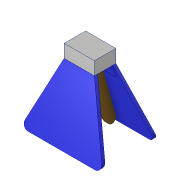
# Autodesk Inventor part: ANTENNA
Saved by Autodesk Inventor 2018 (Build 220112000, 112)
## iProperties
Created: 2020-03-03
Part Number: ANTENNA
Material: Generic
Document SubType Name: Modeling
Designer: nnico
Density: 1 g/cm^3
Appearance: Blue - Wall Paint - Glossy
Author: nnico
Autodesk Inventor part; units mm, degrees
ref_plane "YZ Plane" through (0, 0, 0) normal (1, 0, 0) x (0, 1, 0)
ref_plane "XZ Plane" through (0, 0, 0) normal (0, 1, 0) x (-1, 0, 0)
ref_plane "XY Plane" through (0, 0, 0) normal (0, 0, 1) x (1, 0, 0)
sketch "Sketch1" plane through (0, 0, 0) normal (0, 1, 0) x (-1, 0, 0)
  line L0 (126, -87.5) -> (-126, -87.5)
  line L1 (-126, -87.5) -> (-126, 87.5)
  line L2 (-126, 87.5) -> (126, 87.5)
  line L3 (126, 87.5) -> (126, -87.5)
  line L4 (0, -87.5) -> (0, 87.5) construction
  line L5 (126, 0) -> (-126, 0) construction
  point P0 (0, 0)
  point P1 (0, 0)
  dimension "d0" = 252
  dimension "d1" = 175
  constraints: 12 end point, 5 midpoint, 2 parallel, 1 coincident, 1 horizontal, 1 perpendicular
  measures "d0" distance of L1.end L2.end
  measures "d1" distance of L0.end L1.end
extrude "Extrusion1" add sketch "Sketch1" along normal blind 235
sketch "Sketch3" plane through (0, 235, 0) normal (0, 1, 0) x (1, 0, 0)
  line L0 (126, 87.5) -> (-126, 87.5) projected
  line L1 (-126, 87.5) -> (-126, -87.5) projected
  line L2 (-126, -87.5) -> (126, -87.5) projected
  line L3 (126, -87.5) -> (126, 87.5) projected
  line L4 (-46.5, 33) -> (46.5, 33)
  line L5 (46.5, 33) -> (46.5, -33)
  line L6 (46.5, -33) -> (-46.5, -33)
  line L7 (-46.5, -33) -> (-46.5, 33)
  line L8 (0, 33) -> (0, -33) construction
  line L9 (-46.5, 0) -> (46.5, 0) construction
  point P0 (0, 0)
  point P1 (0, 0)
  dimension "d6" = 93
  dimension "d7" = 66
  constraints: 12 end point, 5 midpoint, 2 parallel, 1 coincident, 1 horizontal, 1 perpendicular
  measures "d6" distance of L5.end L6.end
  measures "d7" distance of L4.end L5.end
extrude "Extrusion2" cut sketch "Sketch3" against normal blind 40
sketch "Sketch4" plane through (-126, 0, 87.5) normal (0, 0, 1) x (1, 0, 0)
  line L0 (79.5, 235) -> (79.5, 195) construction
  line L1 (172.5, 235) -> (172.5, 195) construction
  line L2 (252, 0) -> (0, 0) projected
  line L3 (79.5, 195) -> (0, 0)
  line L4 (172.5, 195) -> (252, 0)
  line L5 (0, 0) -> (0, 195) projected
  line L6 (252, 195) -> (0, 195) projected
  line L7 (252, 0) -> (252, 195) projected
  point P0 (126, 0)
  constraints: 4 end point
extrude "Extrusion3" cut sketch "Sketch4" against normal up to next contours L4 L6 L7 | L5 L6 L3
sketch "Sketch5" plane through (-46.5, 235, -33) normal (-1, 0, 0) x (0, 0, 1)
  line L0 (66, 0) -> (66, -40) projected
  line L1 (120.5, -235) -> (120.5, -40) projected
  line L2 (66, -40) -> (120.5, -235)
  line L3 (120.5, -235) -> (120.5, -40)
  line L4 (120.5, -40) -> (66, -40) projected
  line L5 (120.5, -40) -> (66, -40)
  line L6 (0, -40) -> (-54.5, -40) projected
  line L7 (0, -40) -> (-54.5, -235)
  line L8 (-54.5, -235) -> (-54.5, -40)
  point P0 (33, -235)
  constraints: 10 end point, 2 collinear, 1 vertical
extrude "Extrusion4" cut sketch "Sketch5" along normal up to next
sketch "Sketch6" plane through (-46.5, 235, -33) normal (-1, 0, 0) x (0, 0, 1)
  line L0 (-54.5, -40) -> (0, -40) projected
  line L1 (-54.5, -235) -> (-54.5, -40) projected
  line L2 (-54.5, -235) -> (0, -40) projected
  line L3 (66, -40) -> (120.5, -235) projected
  line L4 (120.5, -40) -> (120.5, -235) projected
  line L5 (66, -40) -> (120.5, -40) projected
  point P0 (33, -235)
extrude "Extrusion5" cut sketch "Sketch6" against normal up to next
sketch "Sketch7" plane through (-46.5, 235, -33) normal (-1, 0, 0) x (0, 0, 1)
  line L0 (66, -40) -> (0, -40) projected
  line L1 (0, -40) -> (10, -40)
  line L2 (0, -40) -> (-54.5, -235) projected
  line L3 (120.5, -235) -> (-54.5, -235) projected
  line L4 (-54.5, -235) -> (-44.5, -235)
  line L5 (-44.5, -235) -> (10, -40)
  line L6 (66, -40) -> (56, -40)
  line L7 (120.5, -235) -> (110.5, -235)
  line L8 (110.5, -235) -> (56, -40)
  line L9 (120.5, -235) -> (66, -40) projected
  point P0 (33, -235)
  dimension "d16" = 10
  dimension "d17" = 10
  dimension "d18" = 10
  dimension "d19" = 10
  constraints: 12 end point, 4 point on line
  measures "d16" distance of L0.end L1.end
  measures "d17" distance of L2.end L4.end
  measures "d18" distance of L0.start L6.end
  measures "d19" distance of L3.start L7.end
extrude "Extrusion6" cut sketch "Sketch7" along normal up to next contours L8 L3 L5 L0
sketch "Sketch8" plane through (-46.5, 235, -33) normal (-1, 0, 0) x (0, 0, 1)
  line L0 (110.5, -235) -> (56, -40) projected
  line L1 (10, -40) -> (-44.5, -235) projected
  line L2 (56, -40) -> (10, -40)
  line L3 (110.5, -235) -> (-44.5, -235) projected
  point P0 (33, -235)
  constraints: 2 end point, 1 horizontal
extrude "Extrusion7" cut sketch "Sketch8" against normal blind 40.5
sketch "Sketch9" plane through (46.5, 235, 33) normal (1, 0, 0) x (0, 0, -1)
  line L0 (10, -40) -> (-44.5, -235) projected
  line L1 (56, -40) -> (10, -40) projected
  line L2 (110.5, -235) -> (56, -40) projected
  line L3 (-44.5, -235) -> (110.5, -235) projected
  point P0 (33, -235)
extrude "Extrusion8" cut sketch "Sketch9" along normal up to next
sketch "Sketch10" plane through (46.5, 235, 33) normal (1, 0, 0) x (0, 0, -1)
  line L0 (0, -40) -> (10, -40) projected
  line L1 (56, -40) -> (10, -40) projected
  line L2 (10, -40) -> (56, -40)
  line L3 (-44.5, -235) -> (10, -40) projected
  line L4 (110.5, -235) -> (-44.5, -235) projected
  line L5 (56, -40) -> (110.5, -235) projected
  point P0 (33, -235)
  constraints: 2 end point, 1 collinear
extrude "Extrusion9" cut sketch "Sketch10" against normal blind 40.5
sketch "Sketch11" plane through (6, 235, 33) normal (1, 0, 0) x (0, 0, -1)
  line L0 (10, -40) -> (56, -40) construction
  line L1 (33, -40) -> (33, -235) construction
  arc A0 (-40.066, -219.1354) -> (-17.9871, -229.946) centre (-28.0274, -222.5) ccw
  line L2 (110.5, -235) -> (-44.5, -235) construction
  line L3 (-44.5, -235) -> (10, -40) construction
  line L4 (-17.9871, -229.946) -> (33, -161.1943) construction
  line L5 (33, -161.1943) -> (33, -40) construction
  spline S0 degree 2 poles (-17.9871, -229.946) (33, -161.1943) (33, -40) knots 1 1 1 2 2 2
  line L6 (-40.066, -219.1354) -> (-44.5, -235)
  line L7 (-28.0274, -235) -> (33, -235)
  line L8 (33, -235) -> (33, -40)
  line L9 (-28.0274, -235) -> (-44.5, -235)
  arc A1 (83.9871, -229.946) -> (106.066, -219.1354) centre (94.0274, -222.5) ccw
  line L10 (83.9871, -229.946) -> (33, -161.1943) construction
  line L11 (33, -161.1943) -> (33, -40) construction
  spline S1 degree 2 poles (83.9871, -229.946) (33, -161.1943) (33, -40) knots 1 1 1 2 2 2
  line L12 (33, -235) -> (94.0274, -235)
  line L13 (110.5, -235) -> (106.066, -219.1354)
  line L14 (56, -40) -> (110.5, -235) projected
  line L15 (94.0274, -235) -> (110.5, -235)
  dimension "d28" = 25
  constraints: 16 end point, 6 point on circle, 6 tangent, 5 collinear, 4 point on line, 3 symmetric about line, 2 centre point, 1 horizontal, 1 midpoint, 1 vertical, 7 other
  measures "d28" diameter of A0
extrude "Extrusion10" cut sketch "Sketch11" against normal up to next
fillet "Fillet1" radius 15 4 edges at (-126, 0, -82.5) (-126, 0, 82.5) (126, 0, 82.5) (126, 0, -82.5)
sketch "Sketch12" plane through (6, 235, 33) normal (1, 0, 0) x (0, 0, -1)
  arc A0 (-40.066, -219.1354) -> (-17.9871, -229.946) centre (-28.0274, -222.5) ccw projected
  spline S0 degree 2 poles (-17.9871, -229.946) (33, -161.1943) (33, -40) knots 0 0 0 1 1 1 projected
  line L0 (10, -40) -> (33, -40) projected
  line L1 (-40.066, -219.1354) -> (10, -40) projected
  arc A1 (83.9871, -229.946) -> (106.066, -219.1354) centre (94.0274, -222.5) ccw projected
  line L2 (56, -40) -> (106.066, -219.1354) projected
  line L3 (33, -40) -> (56, -40) projected
  spline S1 degree 2 poles (33, -40) (33, -161.1943) (83.9871, -229.946) knots 0 0 0 1 1 1 projected
  point P0 (33, -235)
  constraints: 2 other
extrude "Extrusion11" add sketch "Sketch12" against normal blind 12 separate body
sketch "Sketch13" plane through (6, 235, 33) normal (1, 0, 0) x (0, 0, -1)
  arc A0 (-40.066, -219.1354) -> (-17.9871, -229.946) centre (-28.0274, -222.5) ccw projected
  spline S0 degree 2 poles (-17.9871, -229.946) (33, -161.1943) (33, -40) knots 0 0 0 1 1 1 projected
  line L0 (10, -40) -> (33, -40) projected
  line L1 (-40.066, -219.1354) -> (10, -40) projected
  arc A1 (83.9871, -229.946) -> (106.066, -219.1354) centre (94.0274, -222.5) ccw projected
  line L2 (56, -40) -> (106.066, -219.1354) projected
  line L3 (33, -40) -> (56, -40) projected
  spline S1 degree 2 poles (33, -40) (33, -161.1943) (83.9871, -229.946) knots 0 0 0 1 1 1 projected
  point P0 (33, -235)
  constraints: 2 other
extrude "Extrusion12" cut sketch "Sketch13" against normal up to next bodies 1
sketch "Sketch14" plane through (0, 235, 0) normal (0, 1, 0) x (1, 0, 0)
  line L0 (-46.5, 33) -> (-46.5, -33) projected
  line L1 (-46.5, -33) -> (46.5, -33) projected
  line L2 (46.5, -33) -> (46.5, 33) projected
  line L3 (46.5, 33) -> (-46.5, 33) projected
  point P0 (0, 0)
extrude "Extrusion13" cut sketch "Sketch14" against normal up to next bodies 1
sketch "Sketch15" plane through (6, 195, 23) normal (0, 1, 0) x (1, 0, 0)
  line L0 (-52.5, -10) -> (40.5, -10) projected
  line L1 (-52.5, -10) -> (40.5, -10)
  line L2 (40.5, -10) -> (40.5, 56)
  line L3 (40.5, 56) -> (-52.5, 56)
  line L4 (-52.5, 56) -> (-52.5, -10)
  point P0 (-6, 23)
  constraints: 8 end point, 2 parallel, 1 horizontal, 1 perpendicular
extrude "Extrusion14" add sketch "Sketch15" along normal blind 40 separate body
body "Solid1"
body "Solid2"
body "Solid3"
